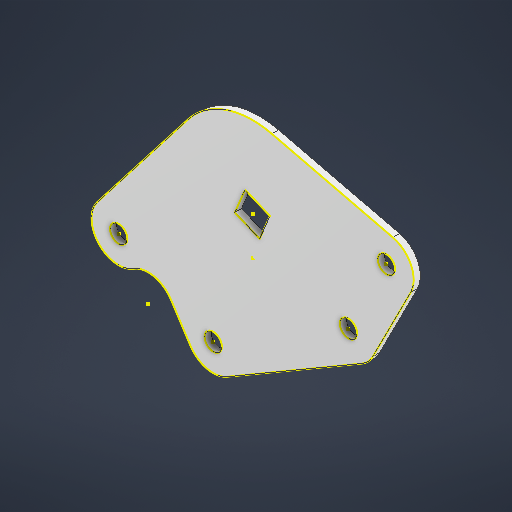
# Autodesk Inventor part: Front Horizontal Odom Pod Rot Side
Saved by Autodesk Inventor 2025 (Build 290162010, 162A)
## iProperties
Created: 2024-11-03
Part Number: Front Horizontal Odom Pod Rot Side
Material: Acetal Resin, White
Document SubType Name: Sheet Metal
Designer: blips
Density: 1.425 g/cm^3
Sheet Metal Rule: Default
Appearance: Smooth - White
Author: blips
Autodesk Inventor part; units mm, degrees
ref_plane "YZ Plane" through (0, 0, 0) normal (1, 0, 0) x (0, 1, 0)
ref_plane "XZ Plane" through (0, 0, 0) normal (0, 1, 0) x (-1, 0, 0)
ref_plane "XY Plane" through (0, 0, 0) normal (0, 0, 1) x (1, 0, 0)
ref_plane "Work Plane1" through (0, 0, 0) normal (0, 0, 1) x (1, 0, 0)
sketch "Sketch1" plane through (0, 0, 0) normal (0, 0, 1) x (1, 0, 0)
  line L0 (1.6592, 4.7063) -> (-4.1605, 7.1169)
  line L1 (-4.1605, 7.1169) -> (-1.7499, 12.9366)
  line L2 (-1.7499, 12.9366) -> (4.0698, 10.526)
  line L3 (4.0698, 10.526) -> (1.6592, 4.7063)
  circle A0 centre (31.2751, 14.3567) radius 2.032
  circle A1 centre (-31.2751, -10.7579) radius 2.032
  circle A2 centre (-9.1964, -21.5433) radius 2.032
  line L4 (4.4799, 27.3609) -> (32.7659, 20.5292)
  arc A3 (4.4799, 27.3609) -> (-15.0435, 20.5211) centre (0.0075, 8.8433) ccw
  line L5 (-36.2921, -6.8653) -> (-15.0435, 20.5211)
  arc A4 (-36.2921, -6.8653) -> (-27.8312, -16.0929) centre (-31.2751, -10.7579) ccw
  arc A5 (-19.0523, -17.9839) -> (-27.8312, -16.0929) centre (-24.3873, -21.4279) ccw
  line L6 (-14.5314, -24.9873) -> (-19.0523, -17.9839)
  arc A6 (36.9334, 11.4747) -> (32.7659, 20.5292) centre (31.2751, 14.3567) ccw
  arc A7 (-14.5314, -24.9873) -> (-5.9915, -27.0252) centre (-9.1964, -21.5433) ccw
  arc A8 (25.6029, -8.5539) -> (28.0563, -5.954) centre (22.398, -3.072) ccw
  circle A9 centre (22.398, -3.072) radius 2.032
  line L7 (36.9334, 11.4747) -> (28.0563, -5.954)
  line L8 (25.6029, -8.5539) -> (-5.9915, -27.0252)
  line L9 (72.5061, 7.5054) -> (72.5061, 11.8054)
  point P0 (0, 0)
  dimension "d14" = 4.064
  measures "d14" diameter of A9
extrude "Plate3" add sketch "Sketch1" along normal blind 1.5875
sketch "Sketch2" plane through (0, 0, 1.5875) normal (0, 0, 1) x (1, 0, 0)
  arc A0 (4.4799, 27.3609) -> (-15.0435, 20.5211) centre (0.0075, 8.8433) ccw projected
  line L0 (4.4799, 27.3609) -> (32.7659, 20.5292) projected
  arc A1 (36.9334, 11.4747) -> (32.7659, 20.5292) centre (31.2751, 14.3567) ccw projected
  line L1 (36.9334, 11.4747) -> (28.0563, -5.954) projected
  arc A2 (25.6029, -8.5539) -> (28.0563, -5.954) centre (22.398, -3.072) ccw projected
  line L2 (25.6029, -8.5539) -> (-5.9915, -27.0252) projected
  arc A3 (-14.5314, -24.9873) -> (-5.9915, -27.0252) centre (-9.1964, -21.5433) ccw projected
  line L3 (-14.5314, -24.9873) -> (-19.0523, -17.9839) projected
  arc A4 (-19.0523, -17.9839) -> (-27.8312, -16.0929) centre (-24.3873, -21.4279) ccw projected
  arc A5 (-36.2921, -6.8653) -> (-27.8312, -16.0929) centre (-31.2751, -10.7579) ccw projected
  line L4 (-36.2921, -6.8653) -> (-15.0435, 20.5211) projected
  line L5 (-1.7499, 12.9366) -> (4.0698, 10.526) projected
  line L6 (-4.1605, 7.1169) -> (-1.7499, 12.9366) projected
  line L7 (1.6592, 4.7063) -> (-4.1605, 7.1169) projected
  line L8 (4.0698, 10.526) -> (1.6592, 4.7063) projected
  circle A6 centre (31.2751, 14.3567) radius 2.032 projected
  circle A7 centre (22.398, -3.072) radius 2.032 projected
  circle A8 centre (-9.1964, -21.5433) radius 2.032 projected
  circle A9 centre (-31.2751, -10.7579) radius 2.032 projected
  point P0 (0, 0)
equation "\"d15\" = Thickness"
equation "\"BendRadius\" = Thickness"
equation "\"BendReliefWidth\" = Thickness"
equation "\"BendReliefDepth\" = 0.5 * Thickness"
equation "\"CornerReliefSize\" = 4 * Thickness"
equation "\"MinimumRemnant\" = 2 * Thickness"
equation "\"TransitionRadius\" = BendRadius"
equation "\"JacobiRadiusSize\" = BendRadius"
equation "\"GapSize\" = Thickness"
equation "\"Thickness\" = 1.5875"
body "Solid3"
